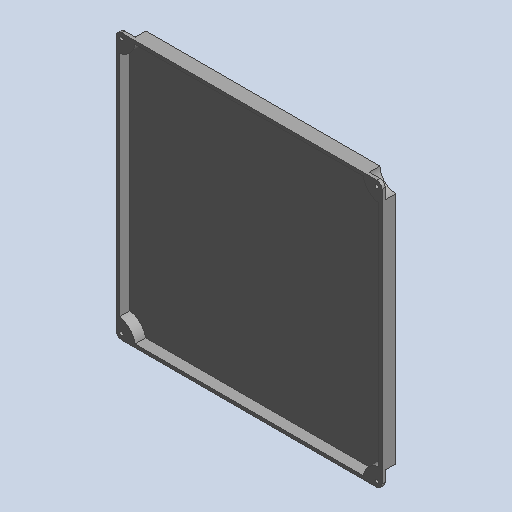
# Autodesk Inventor part: Enclosure cover
Saved by Autodesk Inventor 2026 (Build 300175050, 175E)
## iProperties
Part Number: Enclosure cover
Material: Generic
Document SubType Name: Modeling
Designer: Kartik
Mass: 216.149 g
Surface Area: 1472 cm^2
Volume: 216.149 cm^3
Density: 1 g/cm^3
Appearance: Default
Author: Kartik
Autodesk Inventor part; units mm, degrees
ref_plane "YZ Plane" through (0, 0, 0) normal (1, 0, 0) x (0, 1, 0)
ref_plane "XZ Plane" through (0, 0, 0) normal (0, 1, 0) x (-1, 0, 0)
ref_plane "XY Plane" through (0, 0, 0) normal (0, 0, 1) x (1, 0, 0)
sketch "Sketch1" plane through (0, 0, 0) normal (0, 0, 1) x (1, 0, 0)
  line L0 (-123.0769, 96.9231) -> (96.9231, 96.9231)
  line L1 (111.9231, 81.9231) -> (111.9231, -138.0769)
  line L2 (96.9231, -153.0769) -> (-123.0769, -153.0769)
  line L3 (-138.0769, -138.0769) -> (-138.0769, 81.9231)
  arc A0 (-138.0769, 81.9231) -> (-123.0769, 96.9231) centre (-138.0769, 96.9231) ccw
  arc A1 (96.9231, 96.9231) -> (111.9231, 81.9231) centre (111.9231, 96.9231) ccw
  arc A2 (111.9231, -138.0769) -> (96.9231, -153.0769) centre (111.9231, -153.0769) ccw
  arc A3 (-123.0769, -153.0769) -> (-138.0769, -138.0769) centre (-138.0769, -153.0769) ccw
  point P0 (0, 0)
  dimension "d4" = 30
  dimension "d5" = 30
  dimension "d6" = 30
  dimension "d7" = 30
  dimension "d27" = 250
  dimension "d28" = 250
  constraints: 8 end point, 8 point on circle, 4 centre point, 3 equal length, 2 parallel, 1 horizontal, 1 perpendicular
  measures "d4" diameter of A0
  measures "d5" diameter of A1
  measures "d6" diameter of A2
  measures "d7" diameter of A3
  measures "d27" distance of A1.centre A2.centre
  measures "d28" distance of A0.centre A1.centre
extrude "Extrusion1" add sketch "Sketch1" along normal blind 3
sketch "Sketch2" plane through (0, 0, 3) normal (0, 0, 1) x (1, 0, 0)
  line L0 (-123.0769, -153.0769) -> (96.9231, -153.0769) projected
  arc A0 (111.9231, -138.0769) -> (96.9231, -153.0769) centre (111.9231, -153.0769) ccw projected
  line L1 (111.9231, -138.0769) -> (111.9231, 81.9231) projected
  arc A1 (96.9231, 96.9231) -> (111.9231, 81.9231) centre (111.9231, 96.9231) ccw projected
  line L2 (96.9231, 96.9231) -> (-123.0769, 96.9231) projected
  arc A2 (-138.0769, 81.9231) -> (-123.0769, 96.9231) centre (-138.0769, 96.9231) ccw projected
  line L3 (-138.0769, 81.9231) -> (-138.0769, -138.0769) projected
  arc A3 (-123.0769, -153.0769) -> (-138.0769, -138.0769) centre (-138.0769, -153.0769) ccw projected
  line L4 (-120.3287, 93.9231) -> (94.1748, 93.9231)
  arc A4 (94.1748, 93.9231) -> (108.9231, 79.1748) centre (111.9231, 96.9231) ccw
  line L5 (108.9231, 79.1748) -> (108.9231, -135.3287)
  arc A5 (108.9231, -135.3287) -> (94.1748, -150.0769) centre (111.9231, -153.0769) ccw
  line L6 (94.1748, -150.0769) -> (-120.3287, -150.0769)
  arc A6 (-120.3287, -150.0769) -> (-135.0769, -135.3287) centre (-138.0769, -153.0769) ccw
  line L7 (-135.0769, -135.3287) -> (-135.0769, 79.1748)
  arc A7 (-135.0769, 79.1748) -> (-120.3287, 93.9231) centre (-138.0769, 96.9231) ccw
  point P0 (0, 0)
  dimension "d8" = 3
  constraints: 8 end point, 8 point on circle, 4 centre point, 7 other
  measures "d8" distance between parallel lines of L2 L4
extrude "Extrusion2" add sketch "Sketch2" along normal blind 10
sketch "Sketch3" plane through (0, 0, 13) normal (0, 0, 1) x (1, 0, 0)
  line L0 (96.9231, 96.9231) -> (-123.0769, 96.9231) projected
  line L1 (-138.0769, 81.9231) -> (-138.0769, -138.0769) projected
  line L2 (111.9231, -138.0769) -> (111.9231, 81.9231) projected
  line L3 (-123.0769, -153.0769) -> (96.9231, -153.0769) projected
  arc A0 (111.9231, -138.0769) -> (96.9231, -153.0769) centre (111.9231, -153.0769) ccw projected
  arc A1 (-123.0769, -153.0769) -> (-138.0769, -138.0769) centre (-138.0769, -153.0769) ccw projected
  arc A2 (-138.0769, 81.9231) -> (-123.0769, 96.9231) centre (-138.0769, 96.9231) ccw projected
  arc A3 (96.9231, 96.9231) -> (111.9231, 81.9231) centre (111.9231, 96.9231) ccw projected
  line L4 (-138.0769, 96.9231) -> (111.9231, 96.9231)
  line L5 (111.9231, 96.9231) -> (111.9231, -153.0769)
  line L6 (111.9231, -153.0769) -> (-138.0769, -153.0769)
  line L7 (-138.0769, -153.0769) -> (-138.0769, 96.9231)
  point P0 (0, 0)
  point P1 (106.9231, 96.9231)
  point P2 (-133.0769, 86.9231)
  point P3 (116.9231, -143.0769)
  point P4 (111.9231, -138.0769)
  point P5 (-138.0769, -138.0769)
  point P6 (-123.0769, -153.0769)
  point P7 (-133.0769, 86.9231)
  point P8 (111.9231, 81.9231)
  point P9 (96.9231, 96.9231)
  constraints: 8 end point, 2 parallel, 1 horizontal, 1 perpendicular, 2 other
extrude "Extrusion3" add sketch "Sketch3" against normal blind 3 contours L4 L5 A3 | A2 L7 L4 | L5 L6 A0 | A1 L6 L7
fillet "Fillet1" radius 5 4 edges at (111.9231, -153.0769, 11.5) (-138.0769, -153.0769, 11.5) (111.9231, 96.9231, 11.5) (-138.0769, 96.9231, 11.5)
sketch "Sketch4" plane through (0, 0, 13) normal (0, 0, 1) x (1, 0, 0)
  arc A0 (-133.0769, 96.9231) -> (-138.0769, 91.9231) centre (-133.0769, 91.9231) ccw projected
  line L0 (-138.0769, 91.9231) -> (-138.0769, -148.0769) projected
  arc A1 (-138.0769, -148.0769) -> (-133.0769, -153.0769) centre (-133.0769, -148.0769) ccw projected
  line L1 (-133.0769, -153.0769) -> (106.9231, -153.0769) projected
  arc A2 (106.9231, -153.0769) -> (111.9231, -148.0769) centre (106.9231, -148.0769) ccw projected
  line L2 (111.9231, -148.0769) -> (111.9231, 91.9231) projected
  arc A3 (111.9231, 91.9231) -> (106.9231, 96.9231) centre (106.9231, 91.9231) ccw projected
  line L3 (106.9231, 96.9231) -> (-133.0769, 96.9231) projected
  line L4 (-120.3287, 93.9231) -> (94.1748, 93.9231) projected
  arc A4 (94.1748, 93.9231) -> (108.9231, 79.1748) centre (111.9231, 96.9231) ccw projected
  line L5 (108.9231, 79.1748) -> (108.9231, -135.3287) projected
  arc A5 (108.9231, -135.3287) -> (94.1748, -150.0769) centre (111.9231, -153.0769) ccw projected
  line L6 (94.1748, -150.0769) -> (-120.3287, -150.0769) projected
  arc A6 (-120.3287, -150.0769) -> (-135.0769, -135.3287) centre (-138.0769, -153.0769) ccw projected
  line L7 (-135.0769, -135.3287) -> (-135.0769, 79.1748) projected
  arc A7 (-135.0769, 79.1748) -> (-120.3287, 93.9231) centre (-138.0769, 96.9231) ccw projected
  circle A8 centre (-133.0769, 91.9231) radius 1.6
  circle A9 centre (-133.0769, -148.0769) radius 1.6
  circle A10 centre (106.9231, 91.9231) radius 1.6
  circle A11 centre (106.9231, -148.0769) radius 1.6
  point P0 (0, 0)
  dimension "d14" = 3.2
  dimension "d15" = 5
  dimension "d16" = 5
  dimension "d19" = 240
  dimension "d22" = 240
  constraints: 4 centre point, 1 horizontal, 1 vertical, 6 other
  measures "d14" diameter of A8
  measures "d15" distance from line of L3 A8.centre
  measures "d16" distance from line of A8.centre L0
  measures "d19" distance of A8.centre A9.centre
  measures "d22" distance of A8.centre A10.centre
extrude "Extrusion4" cut sketch "Sketch4" against normal blind 3 contours A8 | A9 | A10 | A11
body "Solid1"
